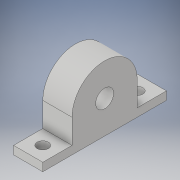
# Autodesk Inventor part: bearingStandin
Saved by Autodesk Inventor 2019 (Build 230136000, 136)
## iProperties
Created: 2019-05-07
Part Number: bearingStandin
Material: Generic
Document SubType Name: Modeling
Designer: Alex Jones
Density: 1 g/cm^3
Appearance: Default
Author: Alex Jones
Autodesk Inventor part; units mm, degrees
ref_plane "YZ Plane" through (0, 0, 0) normal (1, 0, 0) x (0, 1, 0)
ref_plane "XZ Plane" through (0, 0, 0) normal (0, 1, 0) x (-1, 0, 0)
ref_plane "XY Plane" through (0, 0, 0) normal (0, 0, 1) x (1, 0, 0)
sketch "Sketch1" plane through (0, 0, 0) normal (1, 0, 0) x (0, 1, 0)
  line L0 (-1.8333, 27.5) -> (1.8333, 27.5)
  line L1 (1.8333, -27.5) -> (-1.8333, -27.5)
  line L2 (-1.8333, -27.5) -> (-1.8333, 27.5)
  line L3 (-1.8333, 27.5) -> (1.8333, -27.5) construction
  line L4 (1.8333, 27.5) -> (-1.8333, -27.5) construction
  arc A0 (12.6667, -14.5) -> (12.6667, 14.5) centre (12.6667, 0) ccw
  line L5 (12.6667, 14.5) -> (1.8333, 14.5)
  line L6 (12.6667, -14.5) -> (1.8333, -14.5)
  circle A1 centre (12.6667, 0) radius 4
  line L7 (1.8333, 27.5) -> (1.8333, 14.5)
  line L8 (1.8333, -14.5) -> (1.8333, -27.5)
  point P0 (0, 0)
  dimension "d0" = 55
  dimension "d2" = 8
  constraints: 18 end point, 3 horizontal, 3 parallel, 2 centre point, 2 midpoint, 2 perpendicular, 2 point on circle, 2 tangent, 1 coincident
  measures "d0" distance between parallel lines of L1 L0
  measures "d2" diameter of A1
extrude "Extrusion1" add sketch "Sketch1" along normal blind 13
sketch "Sketch2" plane through (0, 1.8333, 27.5) normal (0, 1, 0) x (1, 0, 0)
  line L0 (13, 13) -> (13, 42) projected
  line L1 (0, 0) -> (13, 13) construction
  line L2 (0, 55) -> (0, 0) projected
  line L3 (0, 42) -> (13, 42) projected
  line L4 (0, 55) -> (13, 42) construction
  circle A0 centre (6.5, 6.5) radius 2.5
  circle A1 centre (6.5, 48.5) radius 2.5
  point P0 (0, 27.5)
  dimension "d5" = 5
  dimension "d6" = 5
  constraints: 4 end point, 2 centre point, 2 midpoint
  measures "d5" diameter of A0
  measures "d6" diameter of A1
extrude "Extrusion2" cut sketch "Sketch2" against normal blind 13
body "Solid1"
